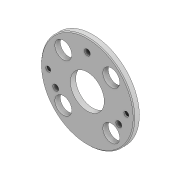
# Autodesk Inventor part: AMT102Mount
Saved by Autodesk Inventor 2021 (Build 250183000, 183)
## iProperties
Created: 2020-08-06
Part Number: AMT102Mount
Material: Generic
Document SubType Name: Modeling
Designer: Derm
Density: 1 g/cm^3
Appearance: Default
Author: Derm
Autodesk Inventor part; units mm, degrees
ref_plane "YZ Plane" through (0, 0, 0) normal (1, 0, 0) x (0, 1, 0)
ref_plane "XZ Plane" through (0, 0, 0) normal (0, 1, 0) x (-1, 0, 0)
ref_plane "XY Plane" through (0, 0, 0) normal (0, 0, 1) x (1, 0, 0)
sketch "Sketch1" plane through (0, 0, 0) normal (0, 0, 1) x (1, 0, 0)
  circle A0 centre (-43.9508, -25.375) radius 1.8 projected
  circle A1 centre (0, -50.75) radius 1.8 projected
  circle A2 centre (43.9508, -25.375) radius 1.8 projected
  circle A3 centre (43.9508, 25.375) radius 1.8 projected
  circle A4 centre (0, 50.75) radius 1.8 projected
  circle A5 centre (-43.9508, 25.375) radius 1.8 projected
  circle A6 centre (0, 0) radius 55 projected
  circle A7 centre (0, 0) radius 10 projected
  line L0 (-5, -45.3652) -> (-5, -28.788) projected
  arc A8 (-3.319, -27.299) -> (-5, -28.788) centre (-3.5, -28.788) ccw projected
  arc A9 (-3.319, -27.299) -> (3.319, -27.299) centre (0, 0) ccw projected
  arc A10 (5, -28.788) -> (3.319, -27.299) centre (3.5, -28.788) ccw projected
  line L1 (5, -28.788) -> (5, -45.3652) projected
  arc A11 (3.6154, -46.8607) -> (5, -45.3652) centre (3.5, -45.3652) ccw projected
  arc A12 (-3.6154, -46.8607) -> (3.6154, -46.8607) centre (0, 0) ccw projected
  arc A13 (-5, -45.3652) -> (-3.6154, -46.8607) centre (-3.5, -45.3652) ccw projected
  arc A14 (3.6154, 46.8607) -> (-3.6154, 46.8607) centre (0, 0) ccw projected
  arc A15 (5, 45.3652) -> (3.6154, 46.8607) centre (3.5, 45.3652) ccw projected
  line L2 (5, 45.3652) -> (5, 28.788) projected
  arc A16 (3.319, 27.299) -> (5, 28.788) centre (3.5, 28.788) ccw projected
  arc A17 (3.319, 27.299) -> (-3.319, 27.299) centre (0, 0) ccw projected
  arc A18 (-5, 28.788) -> (-3.319, 27.299) centre (-3.5, 28.788) ccw projected
  line L3 (-5, 28.788) -> (-5, 45.3652) projected
  arc A19 (-3.6154, 46.8607) -> (-5, 45.3652) centre (-3.5, 45.3652) ccw projected
  circle A20 centre (25.375, -43.9508) radius 3.75 projected
  arc A21 (11.8791, -45.474) -> (23.5, -40.7032) centre (0, 0) ccw projected
  arc A22 (10, -44.0227) -> (11.8791, -45.474) centre (11.5, -44.0227) ccw projected
  line L4 (10, -44.0227) -> (10, -26.6224) projected
  arc A23 (10.9052, -25.2453) -> (10, -26.6224) centre (11.5, -26.6224) ccw projected
  arc A24 (10.9052, -25.2453) -> (25.2453, -10.9052) centre (0, 0) ccw projected
  arc A25 (26.6224, -10) -> (25.2453, -10.9052) centre (26.6224, -11.5) ccw projected
  line L5 (26.6224, -10) -> (44.0227, -10) projected
  arc A26 (45.474, -11.8791) -> (44.0227, -10) centre (44.0227, -11.5) ccw projected
  arc A27 (23.5, -40.7032) -> (45.474, -11.8791) centre (0, 0) ccw projected
  circle A28 centre (-50.75, 0) radius 3.75 projected
  arc A29 (-46.8607, 3.6154) -> (-47, 0) centre (0, 0) ccw projected
  arc A30 (-45.3652, 5) -> (-46.8607, 3.6154) centre (-45.3652, 3.5) ccw projected
  line L6 (-45.3652, 5) -> (-28.788, 5) projected
  arc A31 (-27.299, 3.319) -> (-28.788, 5) centre (-28.788, 3.5) ccw projected
  arc A32 (-27.299, 3.319) -> (-27.299, -3.319) centre (0, 0) ccw projected
  arc A33 (-28.788, -5) -> (-27.299, -3.319) centre (-28.788, -3.5) ccw projected
  line L7 (-28.788, -5) -> (-45.3652, -5) projected
  arc A34 (-46.8607, -3.6154) -> (-45.3652, -5) centre (-45.3652, -3.5) ccw projected
  arc A35 (-47, 0) -> (-46.8607, -3.6154) centre (0, 0) ccw projected
  circle A36 centre (25.375, 43.9508) radius 3.75 projected
  arc A37 (45.474, 11.8791) -> (23.5, 40.7032) centre (0, 0) ccw projected
  arc A38 (44.0227, 10) -> (45.474, 11.8791) centre (44.0227, 11.5) ccw projected
  line L8 (44.0227, 10) -> (26.6224, 10) projected
  arc A39 (25.2453, 10.9052) -> (26.6224, 10) centre (26.6224, 11.5) ccw projected
  arc A40 (25.2453, 10.9052) -> (10.9052, 25.2453) centre (0, 0) ccw projected
  arc A41 (10, 26.6224) -> (10.9052, 25.2453) centre (11.5, 26.6224) ccw projected
  line L9 (10, 26.6224) -> (10, 44.0227) projected
  arc A42 (11.8791, 45.474) -> (10, 44.0227) centre (11.5, 44.0227) ccw projected
  arc A43 (23.5, 40.7032) -> (11.8791, 45.474) centre (0, 0) ccw projected
  circle A44 centre (-25.375, 43.9508) radius 3.75 projected
  arc A45 (-11.8791, 45.474) -> (-23.5, 40.7032) centre (0, 0) ccw projected
  arc A46 (-10, 44.0227) -> (-11.8791, 45.474) centre (-11.5, 44.0227) ccw projected
  line L10 (-10, 44.0227) -> (-10, 26.6224) projected
  arc A47 (-10.9052, 25.2453) -> (-10, 26.6224) centre (-11.5, 26.6224) ccw projected
  arc A48 (-10.9052, 25.2453) -> (-25.2453, 10.9052) centre (0, 0) ccw projected
  arc A49 (-26.6224, 10) -> (-25.2453, 10.9052) centre (-26.6224, 11.5) ccw projected
  line L11 (-26.6224, 10) -> (-44.0227, 10) projected
  arc A50 (-45.474, 11.8791) -> (-44.0227, 10) centre (-44.0227, 11.5) ccw projected
  arc A51 (-23.5, 40.7032) -> (-45.474, 11.8791) centre (0, 0) ccw projected
  circle A52 centre (-25.375, -43.9508) radius 3.75 projected
  arc A53 (-45.474, -11.8791) -> (-23.5, -40.7032) centre (0, 0) ccw projected
  arc A54 (-44.0227, -10) -> (-45.474, -11.8791) centre (-44.0227, -11.5) ccw projected
  line L12 (-44.0227, -10) -> (-26.6224, -10) projected
  arc A55 (-25.2453, -10.9052) -> (-26.6224, -10) centre (-26.6224, -11.5) ccw projected
  arc A56 (-25.2453, -10.9052) -> (-10.9052, -25.2453) centre (0, 0) ccw projected
  arc A57 (-10, -26.6224) -> (-10.9052, -25.2453) centre (-11.5, -26.6224) ccw projected
  line L13 (-10, -26.6224) -> (-10, -44.0227) projected
  arc A58 (-11.8791, -45.474) -> (-10, -44.0227) centre (-11.5, -44.0227) ccw projected
  arc A59 (-23.5, -40.7032) -> (-11.8791, -45.474) centre (0, 0) ccw projected
  circle A60 centre (50.75, 0) radius 3.75 projected
  arc A61 (46.8607, -3.6154) -> (47, 0) centre (0, 0) ccw projected
  arc A62 (45.3652, -5) -> (46.8607, -3.6154) centre (45.3652, -3.5) ccw projected
  line L14 (45.3652, -5) -> (28.788, -5) projected
  arc A63 (27.299, -3.319) -> (28.788, -5) centre (28.788, -3.5) ccw projected
  arc A64 (27.299, -3.319) -> (27.299, 3.319) centre (0, 0) ccw projected
  arc A65 (28.788, 5) -> (27.299, 3.319) centre (28.788, 3.5) ccw projected
  line L15 (28.788, 5) -> (45.3652, 5) projected
  arc A66 (46.8607, 3.6154) -> (45.3652, 5) centre (45.3652, 3.5) ccw projected
  arc A67 (47, 0) -> (46.8607, 3.6154) centre (0, 0) ccw projected
  circle A68 centre (-14.1421, -14.1421) radius 5 projected
  circle A69 centre (14.1421, 14.1421) radius 5 projected
  circle A70 centre (-14.1421, 14.1421) radius 5 projected
  circle A71 centre (14.1421, -14.1421) radius 5 projected
  circle A72 centre (0, 0) radius 27.5
  circle A73 centre (0, 20) radius 1.75 projected
  circle A74 centre (-18.6, -7.3511) radius 1.75 projected
  circle A75 centre (18.6, -7.3512) radius 1.75 projected
  point P0 (0, 0)
  point P1 (-27.299, -3.319)
  point P2 (-25.2453, -10.9052)
  point P3 (-10.9052, -25.2453)
  point P4 (3.319, -27.299)
  point P5 (25.2453, -10.9052)
  point P6 (27.299, 3.319)
  point P7 (25.2453, 10.9052)
  point P8 (10.9052, 25.2453)
  point P9 (-3.319, 27.299)
  point P10 (-25.2453, 10.9052)
  constraints: 2 horizontal alignment, 1 centre point, 1 coincident, 4 other
extrude "Extrusion1" add sketch "Sketch1" along normal blind 3.175 contours A72 A56 A32 A48 A17 A40 A64 A24 A9
sketch "Sketch2" plane through (0, 0, 3.175) normal (0, 0, 1) x (1, 0, 0)
  circle A0 centre (-23.0125, 0) radius 1.435 projected
  circle A1 centre (23.0125, 0) radius 1.435 projected
  point P0 (0, 0)
extrude "Extrusion2" cut sketch "Sketch2" against normal blind 3.175
sketch "Sketch3" plane through (0, 0, 0) normal (0, 0, -1) x (-1, 0, 0)
  circle A0 centre (-23.0125, 0) radius 1.435 projected
  circle A1 centre (23.0125, 0) radius 1.435 projected
  line L0 (-23.0125, 3.1754) -> (-20.2625, 1.5877)
  line L1 (-20.2625, 1.5877) -> (-20.2625, -1.5877)
  line L2 (-20.2625, -1.5877) -> (-23.0125, -3.1754)
  line L3 (-23.0125, -3.1754) -> (-25.7625, -1.5877)
  line L4 (-25.7625, -1.5877) -> (-25.7625, 1.5877)
  line L5 (-25.7625, 1.5877) -> (-23.0125, 3.1754)
  circle A2 centre (23.0125, 0) radius 1.435 projected
  line L6 (23.0125, 3.1754) -> (25.7625, 1.5877)
  line L7 (25.7625, 1.5877) -> (25.7625, -1.5877)
  line L8 (25.7625, -1.5877) -> (23.0125, -3.1754)
  line L9 (23.0125, -3.1754) -> (20.2625, -1.5877)
  line L10 (20.2625, -1.5877) -> (20.2625, 1.5877)
  line L11 (20.2625, 1.5877) -> (23.0125, 3.1754)
  point P0 (0, 0)
  dimension "d4" = 5.5
  dimension "d5" = 5.5
  constraints: 24 end point, 2 coincident, 26 other
  measures "d4" distance between parallel lines of L1 L4
  measures "d5" distance between parallel lines of L7 L10
extrude "Extrusion3" cut sketch "Sketch3" against normal blind 2.4
chamfer "Chamfer1" distance 0.5 angle 45 1 edges at (-25.2453, -10.9052, 3.175)
body "Solid1"
